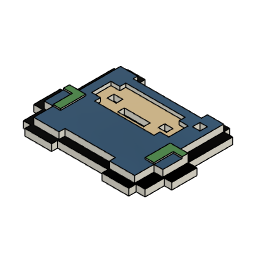
finn v2 (Autodesk Fusion 360 design; units mm, degrees)
Autodesk Fusion 360 part; units mm, degrees
sketch "finn" plane through (0, 0, 0) normal (0, 0, 1) x (1, 0, 0)
  line L0 (12, 6) -> (12, -23)
  line L1 (12, -23) -> (6, -23)
  line L2 (6, -23) -> (6, -41)
  line L3 (6, -41) -> (12, -41)
  line L4 (12, -41) -> (12, -54)
  line L5 (12, -54) -> (17, -54)
  line L6 (17, -58) -> (35, -58)
  line L7 (35, -58) -> (35, -54)
  line L8 (35, -54) -> (69, -54)
  line L9 (69, -58) -> (87, -58)
  line L10 (87, -58) -> (87, -53)
  line L11 (87, -53) -> (93, -53)
  line L12 (93, -53) -> (93, -40)
  line L13 (98, -40) -> (98, -23)
  line L14 (98, -23) -> (92, -23)
  line L15 (92, -23) -> (92, 7)
  line L16 (92, 7) -> (86, 7)
  line L17 (86, 11) -> (74, 11)
  line L18 (74, 11) -> (74, 7)
  line L19 (74, 7) -> (29, 7)
  line L20 (29, 11) -> (17, 11)
  line L21 (17, 11) -> (17, 7)
  line L22 (12, 6) -> (12, 7)
  line L23 (23, -6) -> (23, -19)
  line L24 (23, -19) -> (29, -19)
  line L25 (29, -23) -> (69, -23)
  line L26 (69, -23) -> (69, -19)
  line L27 (75, -19) -> (75, -6)
  line L28 (75, -6) -> (69, -6)
  line L29 (69, -2) -> (69, -6)
  line L30 (69, -2) -> (29, -2)
  line L31 (29, -2) -> (29, -6)
  line L32 (23, -6) -> (29, -6)
  line L33 (29, -10.3517) -> (29, -14.5037)
  line L34 (29, -14.5037) -> (35, -14.5037)
  line L35 (35, -14.5037) -> (35, -10)
  line L36 (35, -10) -> (29, -10)
  line L37 (29, -10) -> (29, -10.3517)
  line L38 (63.4285, -10.1759) -> (69, -10.1759)
  line L39 (69, -10.1759) -> (69, -14.5392)
  line L40 (69, -14.5392) -> (63.393, -14.5392)
  line L41 (63.393, -14.5392) -> (63.4285, -10.1759)
  line L42 (40.5749, -14.5392) -> (40.5749, -19)
  line L43 (40.5749, -19) -> (58, -19)
  line L44 (58, -19) -> (58, -14.5392)
  line L45 (58, -14.5392) -> (40.5749, -14.5392)
  line L46 (17, -58) -> (17, -54)
  line L47 (29, 7) -> (29, 11)
  line L48 (12, 7) -> (17, 7)
  line L49 (12, -23) -> (12, -27)
  line L50 (12, -27) -> (18, -27)
  line L51 (18, -27) -> (18, -40)
  line L52 (18, -40) -> (23, -40)
  line L53 (23, -40) -> (23, -23)
  line L54 (23, -23) -> (12, -23)
  line L55 (92, -23) -> (80, -23)
  line L56 (80, -23) -> (80, -40)
  line L57 (80, -40) -> (86, -40)
  line L58 (86, -40) -> (86, -27)
  line L59 (86, -27) -> (92, -27)
  line L60 (92, -27) -> (92, -23)
  line L61 (69, -58) -> (69, -54)
  line L62 (12, -23) -> (12, -40)
  line L63 (12, -40) -> (18, -40)
  line L64 (18, -53) -> (35, -53)
  line L65 (35, -53) -> (35, -49)
  line L66 (35, -49) -> (69, -49)
  line L67 (69, -53) -> (69, -49)
  line L68 (69, -53) -> (86, -53)
  line L69 (86, -53) -> (86, -40)
  line L70 (86, -40) -> (92, -40)
  line L71 (92, -40) -> (92, -23)
  line L72 (92, -23) -> (86, -23)
  line L73 (92, -23) -> (86, -23)
  line L74 (86, -23) -> (86, 7)
  line L75 (86, 7) -> (75, 7)
  line L76 (75, 7) -> (75, 3)
  line L77 (75, 3) -> (29, 3)
  line L78 (29, 3) -> (29, 6)
  line L79 (29, 6) -> (17.5, 6)
  line L80 (17.5, 6) -> (17.5, -23)
  line L81 (18, -53) -> (18, -40)
  line L82 (93, -40) -> (98, -40)
  line L83 (86, 11) -> (86, 7)
  line L84 (29, -19) -> (29, -23)
  line L85 (69, -19) -> (75, -19)
  line L86 (23, -27) -> (80, -27)
  line L87 (23, -27) -> (23, -40)
  constraint vertical L0
  constraint perpendicular L0 L1
  constraint perpendicular L1 L2
  constraint perpendicular L2 L3
  constraint perpendicular L3 L4
  constraint perpendicular L4 L5
  constraint perpendicular L4 L6
  constraint perpendicular L6 L7
  constraint perpendicular L4 L8
  constraint parallel L8 L9
  constraint perpendicular L9 L10
  constraint perpendicular L10 L11
  constraint perpendicular L11 L12
  constraint perpendicular L11 L13
  constraint perpendicular L13 L14
  constraint perpendicular L11 L15
  constraint perpendicular L15 L16
  constraint perpendicular L15 L17
  constraint perpendicular L17 L18
  constraint perpendicular L18 L19
  constraint perpendicular L18 L20
  constraint perpendicular L20 L21
  constraint parallel L0 L22
  constraint parallel L21 L23
  constraint perpendicular L23 L24
  constraint perpendicular L23 L25
  constraint perpendicular L24 L26
  constraint perpendicular L24 L27
  constraint perpendicular L23 L28
  constraint perpendicular L28 L29
  constraint perpendicular L29 L30
  constraint perpendicular L30 L31
  constraint perpendicular L31 L32
  constraint perpendicular L30 L33
  constraint perpendicular L33 L34
  constraint perpendicular L30 L35
  constraint perpendicular L33 L36
  constraint perpendicular L36 L37
  constraint perpendicular L35 L38
  constraint perpendicular L38 L39
  constraint perpendicular L39 L40
  constraint perpendicular L38 L42
  constraint perpendicular L42 L43
  constraint perpendicular L38 L44
  constraint perpendicular L42 L45
  constraint perpendicular L5 L46
  constraint perpendicular L20 L47
  constraint perpendicular L21 L48
  constraint perpendicular L1 L49
  constraint perpendicular L49 L50
  constraint perpendicular L50 L51
  constraint perpendicular L51 L52
  constraint perpendicular L50 L53
  constraint perpendicular L0 L54
  constraint perpendicular L15 L55
  constraint perpendicular L14 L56
  constraint perpendicular L15 L57
  constraint perpendicular L57 L58
  constraint perpendicular L58 L59
  constraint perpendicular L55 L60
  constraint perpendicular L8 L61
  constraint perpendicular L3 L62
  constraint perpendicular L51 L63
  constraint perpendicular L51 L64
  constraint perpendicular L52 L65
  constraint perpendicular L65 L66
  constraint perpendicular L66 L67
  constraint perpendicular L67 L68
  constraint perpendicular L57 L69
  constraint perpendicular L69 L70
  constraint perpendicular L55 L71
  constraint midpoint L55 L72.end
  constraint perpendicular L16 L74
  constraint perpendicular L74 L75
  constraint perpendicular L75 L76
  constraint perpendicular L76 L77
  constraint perpendicular L77 L78
  constraint perpendicular L78 L79
  constraint midpoint L54 L80.end
  constraint perpendicular L54 L80
  constraint perpendicular L63 L81
  constraint perpendicular L13 L82
  constraint perpendicular L75 L83
  constraint perpendicular L25 L84
  constraint perpendicular L27 L85
  constraint coincident L53 L86.start
  constraint coincident L56 L86.end
  constraint perpendicular L56 L86
  constraint perpendicular L86 L87
extrude "Extrude7" add sketch "finn" along normal blind 10 contours L49 L50 L51 L52 L53 L54 L62 L87 | L55 L56 L57 L58 L59 L60 L71 L72 L73 makes body 1 at (23, -34.3333, 3.3333) makes body 2 at (80, -28.6667, 3.3333)
extrude "Extrude8" add sketch "finn" along normal blind 9 separate body contours L50 L51 L62 L63 | L53 L54 L55 L56 L74 L75 L76 L77 L78 L79 L80 L86 | L52 L53 L56 L57 L64 L65 L66 L67 L68 L69 L81 L86 L87 | L58 L59 L70 L71 makes body 3 at (44.3333, -31.6667, 0)
extrude "Extrude9" add sketch "finn" along normal blind 6.5 contours L23 L24 L25 L26 L27 L28 L29 L30 L31 L32 L84 L85 bodies 3
combine "Combine1" operation add target body 3 tool bodies 1 2
extrude "Extrude10" add sketch "finn" along normal blind 4.5 contours L0 L17 L18 L19 L20 L21 L22 L47 L48 L54 L75 L76 L77 L78 L79 L80 L83 | L1 L2 L3 L4 L5 L6 L7 L8 L9 L10 L11 L12 L13 L14 L46 L49 L60 L61 L62 L63 L64 L65 L66 L67 L68 L69 L70 L71 L81 L82 | L15 L16 L55 L72 L73 L74 bodies 3
extrude "Extrude11" add sketch "finn" along normal blind 2.5 contours L33 L34 L35 L36 L37 | L38 L39 L40 L41 | L42 L43 L44 L45 bodies 3
sketch "Sketch6" plane through (0, 0, 9) normal (0, 0, 1) x (-1, 0, 0)
  line L0 (-23, 19) -> (-23, 6)
  line L1 (-23, 6) -> (-29, 6)
  line L2 (-29, 6) -> (-29, 2)
  line L3 (-29, 2) -> (-69, 2)
  line L4 (-69, 2) -> (-69, 6)
  line L5 (-69, 6) -> (-75, 6)
  line L6 (-75, 6) -> (-75, 19)
  line L7 (-75, 19) -> (-69, 19)
  line L8 (-69, 19) -> (-69, 23)
  line L9 (-69, 23) -> (-29, 23)
  line L10 (-29, 23) -> (-29, 19)
  line L11 (-29, 19) -> (-23, 19)
  line L12 (-23, 23) -> (-23, 40)
  line L13 (-23, 40) -> (-18, 40)
  line L14 (-18, 40) -> (-18, 53)
  line L15 (-18, 53) -> (-35, 53)
  line L16 (-35, 53) -> (-35, 49)
  line L17 (-35, 49) -> (-69, 49)
  line L18 (-69, 49) -> (-69, 53)
  line L19 (-69, 53) -> (-86, 53)
  line L20 (-86, 53) -> (-86, 40)
  line L21 (-86, 40) -> (-80, 40)
  line L22 (-80, 40) -> (-80, 23)
  line L23 (-80, 23) -> (-86, 23)
  line L24 (-86, 23) -> (-86, -7)
  line L25 (-86, -7) -> (-75, -7)
  line L26 (-75, -7) -> (-75, -3)
  line L27 (-75, -3) -> (-29, -3)
  line L28 (-29, -3) -> (-29, -6)
  line L29 (-29, -6) -> (-17.5, -6)
  line L30 (-17.5, -6) -> (-17.5, 23)
  line L31 (-17.5, 23) -> (-23, 23)
  line L32 (-77, 0) -> (-82, 0)
  line L33 (-82, 0) -> (-82, 5)
  line L34 (-82, 5) -> (-77, 5)
  line L35 (-77, 5) -> (-77, 0)
  constraint horizontal L32
  constraint vertical L33
  constraint horizontal L34
  constraint vertical L35
extrude "Extrude13" cut sketch "Sketch6" against normal blind 10 contours L32 L33 L34 L35 bodies 3
named bodies: "finn"
